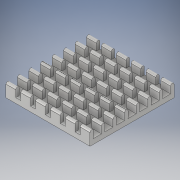
# Autodesk Inventor part: Copper Radiator
Saved by Autodesk Inventor 2019.2 (Build 232265000, 265)
## iProperties
Created: 2018-12-13
Part Number: Copper Radiator
Material: Aluminum 6061-AHC
Document SubType Name: Modeling
Designer: Petar
Density: 2.7 g/cm^3
Appearance: Aluminum - Dark
Author: Petar
Autodesk Inventor part; units mm, degrees
ref_plane "YZ Plane" through (0, 0, 0) normal (1, 0, 0) x (0, 1, 0)
ref_plane "XZ Plane" through (0, 0, 0) normal (0, 1, 0) x (-1, 0, 0)
ref_plane "XY Plane" through (0, 0, 0) normal (0, 0, 1) x (1, 0, 0)
sketch "Sketch1" plane through (0, 0, 0) normal (0, 1, 0) x (-1, 0, 0)
  line L0 (12.5, 12.5) -> (-12.5, 12.5)
  line L1 (-12.5, 12.5) -> (-12.5, -12.5)
  line L2 (-12.5, -12.5) -> (12.5, -12.5)
  line L3 (12.5, -12.5) -> (12.5, 12.5)
  line L4 (0, 12.5) -> (0, -12.5) construction
  line L5 (12.5, 0) -> (-12.5, 0) construction
  point P0 (0, 0)
  point P1 (0, 0)
  dimension "d0" = 25
  dimension "d1" = 25
  constraints: 12 end point, 5 midpoint, 2 parallel, 1 coincident, 1 horizontal, 1 perpendicular
  measures "d0" distance of L2.end L1.end
  measures "d1" distance of L1.end L0.end
extrude "Extrusion1" add sketch "Sketch1" along normal blind 4
sketch "Sketch2" plane through (-12.5, 0, -12.5) normal (-1, 0, 0) x (0, 0, 1)
  line L0 (0, 0) -> (25, 0) projected
  line L1 (0, 0) -> (0, 4) projected
  line L2 (25, 4) -> (0, 4) projected
  line L3 (1, 4) -> (3.42, 4)
  line L4 (3.42, 4) -> (3.42, 1.5)
  line L5 (3.42, 1.5) -> (1, 1.5)
  line L6 (1, 1.5) -> (1, 4)
  line L7 (12.5, 0) -> (12.5, 4) construction
  line L8 (4.42, 4) -> (6.84, 4)
  line L9 (6.84, 4) -> (6.84, 1.5)
  line L10 (6.84, 1.5) -> (4.42, 1.5)
  line L11 (4.42, 1.5) -> (4.42, 4)
  line L12 (7.84, 4) -> (10.26, 4)
  line L13 (10.26, 4) -> (10.26, 1.5)
  line L14 (10.26, 1.5) -> (7.84, 1.5)
  line L15 (7.84, 1.5) -> (7.84, 4)
  line L16 (11.26, 4) -> (13.68, 4)
  line L17 (13.68, 4) -> (13.68, 1.5)
  line L18 (13.68, 1.5) -> (11.26, 1.5)
  line L19 (11.26, 1.5) -> (11.26, 4)
  line L20 (24, 4) -> (21.58, 4)
  line L21 (21.58, 4) -> (21.58, 1.5)
  line L22 (21.58, 1.5) -> (24, 1.5)
  line L23 (24, 1.5) -> (24, 4)
  line L24 (20.58, 4) -> (18.16, 4)
  line L25 (18.16, 4) -> (18.16, 1.5)
  line L26 (18.16, 1.5) -> (20.58, 1.5)
  line L27 (20.58, 1.5) -> (20.58, 4)
  line L28 (17.16, 4) -> (14.74, 4)
  line L29 (14.74, 4) -> (14.74, 1.5)
  line L30 (14.74, 1.5) -> (17.16, 1.5)
  line L31 (17.16, 1.5) -> (17.16, 4)
  line L32 (13.68, 4) -> (11.32, 4)
  line L33 (11.32, 1.5) -> (13.68, 1.5)
  point P0 (13.74, 4)
  point P1 (13.74, 1.5)
  dimension "d5" = 1
  dimension "d6" = 2.42
  dimension "d7" = 2.42
  dimension "d8" = 1
  dimension "d9" = 2.42
  dimension "d10" = 1
  dimension "d12" = 1.5
  dimension "d13" = 2.42
  dimension "d14" = 1
  constraints: 62 end point, 16 symmetric about line, 8 parallel, 6 point on line, 4 horizontal, 4 perpendicular, 2 collinear, 1 midpoint
  measures "d5" distance between parallel lines of L1 L6
  measures "d6" distance of L9.end L10.end
  measures "d7" distance of L13.end L14.end
  measures "d8" distance between parallel lines of L4 L11
  measures "d9" distance of L4.end L5.end
  measures "d10" distance between parallel lines of L9 L15
  measures "d12" distance between parallel lines of L0 L5
  measures "d13" distance of L17.end L18.end
  measures "d14" distance between parallel lines of L19 L13
extrude "Extrusion4" cut sketch "Sketch2" against normal through all
fillet "Fillet1" radius 0.5 16 edges at (0, 4, -12.5) (0, 4, -11.5) (0, 4, -9.08) (0, 4, -8.08) (0, 4, -5.66) (0, 4, -4.66) (0, 4, -2.24) (0, 4, -1.24) (0, 4, 1.18) (0, 4, 2.24) (0, 4, 4.66) (0, 4, 5.66) (0, 4, 8.08) (0, 4, 9.08) (0, 4, 11.5) (0, 4, 12.5)
sketch "Sketch3" plane through (-12.5, 0, 12.5) normal (0, 0, 1) x (1, 0, 0)
  line L0 (0, 0) -> (0, 3.5) projected
  line L1 (0, 0) -> (25, 0) projected
  line L2 (25, 0) -> (25, 3.5) projected
  line L3 (25, 4) -> (0, 4) projected
  line L4 (0, 3.5) -> (0, 4) projected
  line L5 (25, 4) -> (25, 3.5) projected
  line L6 (25, 4) -> (0, 4) projected
  line L7 (2.9167, 4) -> (4.4167, 4)
  line L8 (4.4167, 4) -> (4.4167, 1.5)
  line L9 (4.4167, 1.5) -> (2.9167, 1.5)
  line L10 (2.9167, 1.5) -> (2.9167, 4)
  line L11 (7.3334, 4) -> (8.8334, 4)
  line L12 (8.8334, 1.5) -> (7.3334, 1.5)
  line L13 (7.3334, 1.5) -> (7.3334, 4)
  line L14 (8.8334, 4) -> (8.8334, 1.5)
  line L15 (11.7501, 4) -> (13.2501, 4)
  line L16 (13.2501, 1.5) -> (11.7501, 1.5)
  line L17 (11.7501, 1.5) -> (11.7501, 4)
  line L18 (13.2501, 4) -> (13.2501, 1.5)
  line L19 (16.1668, 4) -> (17.6668, 4)
  line L20 (17.6668, 1.5) -> (16.1668, 1.5)
  line L21 (16.1668, 1.5) -> (16.1668, 4)
  line L22 (17.6668, 4) -> (17.6668, 1.5)
  line L23 (20.5835, 4) -> (22.0835, 4)
  line L24 (22.0835, 1.5) -> (20.5835, 1.5)
  line L25 (20.5835, 1.5) -> (20.5835, 4)
  line L26 (22.0835, 4) -> (22.0835, 1.5)
  point P0 (12.5, 0)
  dimension "d25" = 2.9167
  dimension "d26" = 1.5
  dimension "d27" = 1.5
  dimension "d30" = 4.4167
  dimension "d35" = 2.9165
  constraints: 40 end point, 2 horizontal, 2 parallel, 1 perpendicular, 1 point on line, 32 other
  measures "d25" distance between parallel lines of L10 L0
  measures "d26" distance between parallel lines of L1 L9
  measures "d27" distance between parallel lines of L8 L10
  measures "d30" distance of L7.start L11.start
  measures "d35" distance between parallel lines of L2 L26
extrude "Extrusion5" cut sketch "Sketch3" against normal through all contours L3 L8 L9 L10 | L26 L24 L25 L3 | L3 L14 L12 L13 | L22 L20 L21 L3 | L3 L18 L16 L17
body "Solid1"
